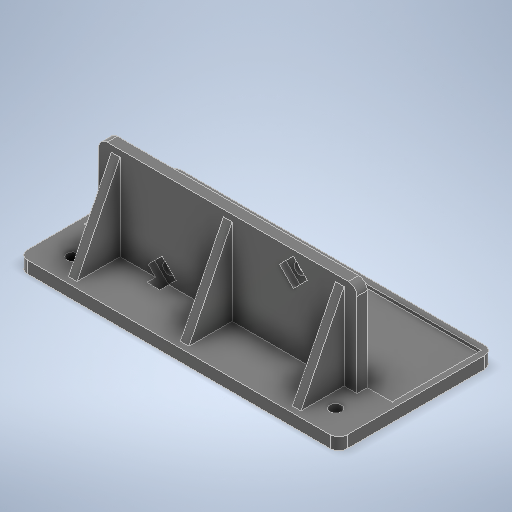
# Autodesk Inventor part: Splitter Mount
Saved by Autodesk Inventor 2025 (Build 290162000, 162)
## iProperties
Created: 2025-03-12
Part Number: Splitter Mount
Material: Plastic, Opaque Black
Document SubType Name: Modeling
Designer: Caleb Fangmeier
Density: 0.952 g/cm^3
Appearance: Smooth - Black
Author: Caleb Fangmeier
Autodesk Inventor part; units mm, degrees
ref_plane "YZ Plane" through (0, 0, 0) normal (1, 0, 0) x (0, 1, 0)
ref_plane "XZ Plane" through (0, 0, 0) normal (0, 1, 0) x (-1, 0, 0)
ref_plane "XY Plane" through (0, 0, 0) normal (0, 0, 1) x (1, 0, 0)
sketch "Sketch1" plane through (0, 0, 0) normal (0, 1, 0) x (-1, 0, 0)
  line L0 (-92.9, 44.9) -> (92.9, 44.9)
  line L1 (92.9, 44.9) -> (92.9, -44.9)
  line L2 (92.9, -44.9) -> (-92.9, -44.9)
  line L3 (-92.9, -44.9) -> (-92.9, 44.9)
  line L4 (-92.9, 44.9) -> (92.9, -44.9) construction
  line L5 (92.9, 44.9) -> (-92.9, -44.9) construction
  point P0 (0, 0)
  dimension "d0" = 185.8
  dimension "d1" = 89.8
  constraints: 12 end point, 2 midpoint, 2 parallel, 1 horizontal, 1 perpendicular
  measures "d0" distance of L1.end L2.end
  measures "d1" distance of L0.end L1.end
extrude "Extrusion1" add sketch "Sketch1" along normal blind 7
sketch "Sketch2" plane through (0, 7, 0) normal (0, 1, 0) x (1, 0, 0)
  line L0 (89.4, -10.4) -> (-89.4, -10.4)
  line L1 (-89.4, -10.4) -> (-89.4, 41.4)
  line L2 (-89.4, 41.4) -> (89.4, 41.4)
  line L3 (89.4, 41.4) -> (89.4, -10.4)
  line L4 (89.4, -10.4) -> (-89.4, 41.4) construction
  line L5 (-89.4, -10.4) -> (89.4, 41.4) construction
  line L6 (92.9, 44.9) -> (-92.9, 44.9) projected
  point P0 (0, 0)
  point P1 (0, 15.5)
  dimension "d4" = 178.8
  dimension "d6" = 51.8
  dimension "d7" = 3.5
  constraints: 12 end point, 2 midpoint, 2 parallel, 1 horizontal, 1 perpendicular, 1 vertical alignment
  measures "d4" distance of L0.start L0.end
  measures "d6" distance of L0.end L1.end
  measures "d7" distance between parallel lines of L6 L2
extrude "Extrusion2" cut sketch "Sketch2" against normal blind 2
sketch "Sketch3" plane through (0, 7, 0) normal (0, 1, 0) x (1, 0, 0)
  line L0 (89.4, -10.4) -> (-89.4, -10.4) projected
  line L1 (75, -10.4) -> (-75, -10.4)
  line L2 (-75, -10.4) -> (-75, -16.4)
  line L3 (-75, -16.4) -> (75, -16.4)
  line L4 (75, -16.4) -> (75, -10.4)
  point P0 (0, 0)
  dimension "d10" = 150
  dimension "d11" = 75
  dimension "d12" = 6
  constraints: 8 end point, 2 parallel, 1 horizontal, 1 perpendicular, 1 point on line
  measures "d10" distance of L2.end L3.end
  measures "d11" distance from line of L2 point (0, 0)
  measures "d12" distance of L1.end L2.end
extrude "Extrusion3" add sketch "Sketch3" along normal blind 53.8
sketch "Sketch4" plane through (-75, 7, 16.4) normal (0, 0, 1) x (1, 0, 0)
  line L0 (150, 0) -> (150, 53.8) projected
  line L1 (0, 53.8) -> (150, 53.8) projected
  line L2 (-14.4, -2) -> (164.4, -2) projected
  line L3 (164.4, -2) -> (-14.4, -2) projected
  point P0 (75, -7)
  point P1 (113.1, 42.45)
  point P2 (36.9, 4.35)
  dimension "d15" = 36.9
  dimension "d17" = 76.2
  dimension "d18" = 38.1
  dimension "d32" = 6.35
  measures "d15" distance from line of L0 point (113.1, 42.45)
  measures "d17" horizontal distance of point (36.9, 4.35) point (113.1, 42.45)
  measures "d18" vertical distance of point (36.9, 4.35) point (113.1, 42.45)
  measures "d32" distance from line of L2 point (36.9, 4.35)
hole "Hole1" at (38.1, 49.45, 16.4) at (-38.1, 11.35, 16.4) direction (0, 0, -1) diameter 6.756 depth 19.05 tip angle 118 clearance for "Socket Head Cap Screw" size "1/4" standard "Ansi Unified Screw Threads"
sketch "Sketch5" plane through (-75, 7, 16.4) normal (0, 0, 1) x (1, 0, 0)
  circle A0 centre (36.9, 4.35) radius 3.378 projected
  line L0 (28.8178, 4.35) -> (36.9, 12.4322)
  line L1 (36.9, 12.4322) -> (44.9822, 4.35)
  line L2 (44.9822, 4.35) -> (36.9, -3.7322)
  line L3 (36.9, -3.7322) -> (28.8178, 4.35)
  line L4 (28.8178, 4.35) -> (44.9822, 4.35) construction
  line L5 (36.9, 12.4322) -> (36.9, -3.7322) construction
  line L6 (28.8178, 4.35) -> (40.2478, 4.35) construction
  circle A1 centre (113.1, 42.45) radius 3.378 projected
  line L7 (105.0178, 42.45) -> (113.1, 50.5322)
  line L8 (113.1, 50.5322) -> (121.1822, 42.45)
  line L9 (121.1822, 42.45) -> (113.1, 34.3678)
  line L10 (113.1, 34.3678) -> (105.0178, 42.45)
  circle A2 centre (113.1, 42.45) radius 3.378 projected
  line L11 (105.0178, 42.45) -> (121.1822, 42.45) construction
  line L12 (113.1, 50.5322) -> (113.1, 34.3678) construction
  line L13 (105.0178, 42.45) -> (116.4478, 42.45) construction
  point P0 (75, -7)
  dimension "d26" = 11.43
  dimension "d27" = 45
  dimension "d28" = 11.43
  dimension "d29" = 11.43
  dimension "d30" = 45
  dimension "d31" = 11.43
  constraints: 28 end point, 4 midpoint, 4 parallel, 2 equal length, 2 horizontal, 2 perpendicular
  measures "d26" distance of L0.start L0.end
  measures "d27" angle of L6 L0
  measures "d28" distance of L0.end L1.end
  measures "d29" distance of L7.start L7.end
  measures "d30" angle of L13 L7
  measures "d31" distance of L7.end L8.end
extrude "Extrusion4" cut sketch "Sketch5" along normal blind 5.08 and the other way blind 3.81
sketch "Sketch6" plane through (0, 0, 0) normal (1, 0, 0) x (0, 1, 0)
  line L0 (7, 16.4) -> (60.8, 16.4) projected
  line L1 (57, 16.4) -> (7, 41.4)
  line L2 (7, -44.9) -> (7, 44.9) projected
  line L3 (7, 44.9) -> (7, -44.9) projected
  line L4 (7, 16.4) -> (7, 21.48) projected
  line L5 (7, 21.48) -> (7, 16.4) projected
  line L6 (7, 16.4) -> (7, 10.4) projected
  line L7 (7, 10.4) -> (7, -41.4) projected
  line L8 (7, -41.4) -> (7, 10.4) projected
  line L9 (7, 10.4) -> (7, 16.4) projected
  point P0 (0, 0)
  dimension "d37" = 50
  dimension "d38" = 25
  constraints: 2 end point, 2 point on line
  measures "d37" distance of L0.start L1.start
  measures "d38" distance from line of L0 L1.end
extrude "Rib1" add sketch "Sketch6" along normal mid plane 5 rib yes fills toward (31.9776, 28.8553) open curves L1
pattern_linear "Rectangular Pattern1" count 3 spacing 65 along (1, 0, 0) of "Rib1" first direction both ways yes
sketch "Sketch7" plane through (0, 7, 0) normal (0, 1, 0) x (1, 0, 0)
  point P0 (0, 0)
  point P1 (76.2, -30)
  point P2 (-76.2, -30)
  dimension "d48" = 76.2
  dimension "d49" = 76.2
  dimension "d50" = 30
  constraints: 1 horizontal alignment
  measures "d48" horizontal distance of point (0, 0) point (76.2, -30)
  measures "d49" horizontal distance of point (0, 0) point (-76.2, -30)
  measures "d50" vertical distance of point (0, 0) point (76.2, -30)
hole "Hole2" at (76.2, 7, 30) at (-76.2, 7, 30) direction (0, -1, 0) diameter 6.756 depth 19.05 tip angle 118 clearance for "Socket Head Cap Screw" size "1/4" standard "Ansi Unified Screw Threads"
fillet "Fillet1" radius 5 6 edges at (-92.9, 3.5, 44.9) (92.9, 3.5, 44.9) (75, 60.8, 13.4) (-75, 60.8, 13.4) (-92.9, 3.5, -44.9) (92.9, 3.5, -44.9)
equation "\"d11\" = 0.5 * d10"
equation "\"d49\" = d48"
body "Solid1"
